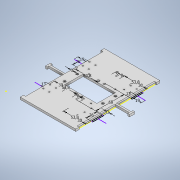
# Autodesk Inventor part: maze_03
Saved by Autodesk Inventor 2020 (Build 240168000, 168)
## iProperties
Created: 2022-07-14
Part Number: maze_03
Material: Типовые
Document SubType Name: Modeling
Designer: akapu
Density: 1 g/cm^3
Appearance: По умолчанию
Author: akapu
Autodesk Inventor part; units mm, degrees
ref_plane "YZ Plane" through (0, 0, 0) normal (1, 0, 0) x (0, 1, 0)
ref_plane "XZ Plane" through (0, 0, 0) normal (0, 1, 0) x (-1, 0, 0)
ref_plane "XY Plane" through (0, 0, 0) normal (0, 0, 1) x (1, 0, 0)
sketch "Эскиз2" plane through (0, 0, 0) normal (0, 1, 0) x (-1, 0, 0)
  line L0 (-166, 0) -> (-166, -200)
  line L1 (-34, 0) -> (-34, -200)
  line L2 (-34, -8) -> (-34, -4)
  line L3 (-9, -53) -> (-196, -53)
  line L4 (-9, -147) -> (-196, -147)
  line L5 (-37, -8) -> (-37, -98)
  line L6 (-37, -98) -> (-29, -98)
  line L7 (-29, -102) -> (-37, -102)
  line L8 (-37, -102) -> (-37, -192)
  line L9 (-166, -192) -> (-163, -192)
  line L10 (-163, -192) -> (-163, -102)
  line L11 (-163, -102) -> (-166, -102)
  line L12 (-166, -102) -> (-166, -192)
  line L13 (-166, -8) -> (-163, -8)
  line L14 (-163, -8) -> (-163, -98)
  line L15 (-163, -98) -> (-166, -98)
  line L16 (-166, -98) -> (-166, -8)
  line L17 (-166, -98) -> (-196, -98)
  line L18 (-196, -98) -> (-196, -102)
  line L19 (-196, -102) -> (-166, -102)
  line L20 (-166, -102) -> (-166, -98)
  line L21 (-29, -98) -> (-4, -98)
  line L22 (-4, -98) -> (-4, -102)
  line L23 (-4, -102) -> (-29, -102)
  line L24 (-29, -102) -> (-29, -98)
  line L25 (-37, -192) -> (-34, -192)
  line L26 (-37, -8) -> (-34, -8)
  line L27 (-4, -102) -> (-4, -106)
  line L28 (-196, -102) -> (-196, -106)
  line L29 (-4, -106) -> (0, -106)
  line L30 (0, -106) -> (0, -94)
  line L31 (0, -94) -> (-4, -94)
  line L32 (-4, -94) -> (-4, -106)
  line L33 (-196, -106) -> (-200, -106)
  line L34 (-200, -106) -> (-200, -94)
  line L35 (-200, -94) -> (-196, -94)
  line L36 (-196, -94) -> (-196, -106)
  line L37 (-34, -200) -> (-166, -200)
  line L38 (-166, 0) -> (-34, 0)
  point P0 (-34, -102)
  point P1 (-34, -98)
  point P2 (-4, -98)
  dimension "d25" = 8
  dimension "d27" = 3
  dimension "d145" = 4
  dimension "d146" = 12
  constraints: 78 end point, 14 parallel, 9 perpendicular, 7 horizontal, 7 point on line, 2 vertical
  measures "d25" distance of L6.end L5.end
  measures "d27" distance of L11.end L10.end
  measures "d145" distance of L22.end L27.end
  measures "d146" distance of L30.end L29.end
extrude "Выдавливание1" add sketch "Эскиз2" along normal blind 5 contours L38 L1 L26 L5 L3 L14 L13 L0 | L15 L14 L3 L5 L6 L1 L7 L8 L4 L10 L11 L0 | L0 L19 L18 L17 | L18 L28 L33 L34 L35 L36 | L6 L24 L7 L1 | L9 L10 L4 L8 L25 L1 L37 L0 | L21 L22 L23 L24 | L32 L31 L30 L29 L27 L22
sketch "Эскиз3" plane through (0, 5, 0) normal (0, 1, 0) x (1, 0, 0)
  line L0 (37, 192) -> (37, 102) projected
  line L1 (37, 147) -> (163, 147)
  line L2 (163, 102) -> (163, 192) projected
  line L3 (37, 98) -> (37, 8) projected
  line L4 (37, 53) -> (163, 53)
  line L5 (163, 147) -> (156, 147)
  line L6 (156, 147) -> (142, 147)
  line L7 (142, 147) -> (142, 155)
  line L8 (142, 155) -> (156, 155)
  line L9 (156, 155) -> (156, 139)
  line L10 (156, 139) -> (142, 139)
  line L11 (142, 139) -> (142, 155)
  line L12 (37, 147) -> (44, 147)
  line L13 (44, 147) -> (58, 147)
  line L14 (58, 147) -> (58, 155)
  line L15 (58, 155) -> (44, 155)
  line L16 (44, 155) -> (44, 139)
  line L17 (44, 139) -> (58, 139)
  line L18 (58, 139) -> (58, 155)
  line L19 (163, 53) -> (156, 53)
  line L20 (156, 53) -> (142, 53)
  line L21 (142, 53) -> (142, 61)
  line L22 (142, 61) -> (58, 61)
  line L23 (58, 61) -> (44, 61)
  line L24 (44, 61) -> (44, 45)
  line L25 (44, 45) -> (58, 45)
  line L26 (58, 45) -> (58, 61)
  line L27 (142, 61) -> (156, 61)
  line L28 (156, 61) -> (156, 45)
  line L29 (156, 45) -> (142, 45)
  line L30 (142, 45) -> (142, 61)
  circle A0 centre (156, 61) radius 1.5
  circle A1 centre (156, 45) radius 1.5
  circle A2 centre (142, 45) radius 1.5
  circle A3 centre (142, 61) radius 1.5
  circle A4 centre (58, 61) radius 1.5
  circle A5 centre (58, 45) radius 1.5
  circle A6 centre (44, 61) radius 1.5
  circle A7 centre (44, 45) radius 1.5
  circle A8 centre (142, 139) radius 1.5
  circle A9 centre (156, 139) radius 1.5
  circle A10 centre (156, 155) radius 1.5
  circle A11 centre (142, 155) radius 1.5
  circle A12 centre (58, 155) radius 1.5
  circle A13 centre (44, 155) radius 1.5
  circle A14 centre (58, 139) radius 1.5
  circle A15 centre (44, 139) radius 1.5
  point P0 (0, 0)
  point P1 (142, 46.5)
  point P2 (143.5, 45)
  dimension "d30" = 7
  dimension "d31" = 14
  dimension "d32" = 8
  dimension "d33" = 16
  dimension "d34" = 7
  dimension "d35" = 14
  dimension "d36" = 8
  dimension "d37" = 16
  dimension "d38" = 7
  dimension "d39" = 14
  dimension "d40" = 8
  dimension "d41" = 16
  dimension "d42" = 16
  dimension "d43" = 3
  dimension "d44" = 3
  dimension "d45" = 3
  dimension "d46" = 3
  dimension "d47" = 3
  dimension "d48" = 3
  dimension "d49" = 3
  dimension "d50" = 3
  dimension "d51" = 3
  dimension "d52" = 3
  dimension "d53" = 3
  dimension "d54" = 3
  dimension "d55" = 3
  dimension "d56" = 3
  dimension "d57" = 3
  dimension "d58" = 3
  constraints: 56 end point, 16 centre point, 16 coincident, 8 parallel, 8 perpendicular, 6 point on line, 5 horizontal, 3 midpoint
  measures "d30" distance of L1.end L5.end
  measures "d31" distance of L5.end L6.end
  measures "d32" distance of L6.end L7.end
  measures "d33" distance of L8.end L9.end
  measures "d34" distance of L1.start L12.end
  measures "d35" distance of L12.end L13.end
  measures "d36" distance of L13.end L14.end
  measures "d37" distance of L16.end L15.end
  measures "d38" distance of L4.end L19.end
  measures "d39" distance of L19.end L20.end
  measures "d40" distance of L20.end L21.end
  measures "d41" distance of L24.end L23.end
  measures "d42" distance of L27.end L28.end
  measures "d43" diameter of A0
  measures "d44" diameter of A1
  measures "d45" diameter of A2
  measures "d46" diameter of A3
  measures "d47" diameter of A4
  measures "d48" diameter of A5
  measures "d49" diameter of A6
  measures "d50" diameter of A7
  measures "d51" diameter of A8
  measures "d52" diameter of A9
  measures "d53" diameter of A10
  measures "d54" diameter of A11
  measures "d55" diameter of A12
  measures "d56" diameter of A13
  measures "d57" diameter of A14
  measures "d58" diameter of A15
extrude "Выдавливание2" cut sketch "Эскиз3" against normal blind 5 contours A13 L15 L16 | L16 L15 A13 | A15 L17 L16 | L16 L17 A15 | A12 L15 L14 | L14 L15 A12 | A14 L17 L18 | L18 L17 A14 | A11 L8 L7 | L7 L8 A11 | A8 L10 L11 | L11 L10 A8 | A10 L8 L9 | L9 L8 A10 | A9 L10 L9 | L9 L10 A9 | A3 L22 L21 | L21 L27 A3 | A2 L29 L30 | L30 L29 A2 | A0 L27 L28 | L28 L27 A0 | A1 L29 L28 | L28 L29 A1 | A5 L25 L26 | L26 L25 A5 | A4 L23 L26 | L26 L22 A4 | L22 A3 L27 | A6 L23 L24 | L24 L23 A6 | A7 L25 L24 | L24 L25 A7 | L23 A4 L22
fillet "Сопряжение1" radius 2 4 edges at (163, 5, -53) (163, 5, -147) (37, 5, -147) (37, 5, -53)
sketch "Эскиз4" plane through (0, 0, 0) normal (0, -1, 0) x (1, 0, 0)
  circle A0 centre (156, -45) radius 1.5 projected
  circle A1 centre (142, -61) radius 1.5 projected
  line L0 (156, -45) -> (142, -45)
  line L1 (142, -45) -> (142, -61)
  line L2 (142, -61) -> (156, -61)
  line L3 (156, -61) -> (156, -45)
  circle A2 centre (156, -139) radius 1.5 projected
  circle A3 centre (142, -155) radius 1.5 projected
  line L4 (156, -139) -> (142, -139)
  line L5 (142, -139) -> (142, -155)
  line L6 (142, -155) -> (156, -155)
  line L7 (156, -155) -> (156, -139)
  circle A4 centre (58, -139) radius 1.5 projected
  circle A5 centre (44, -155) radius 1.5 projected
  line L8 (58, -139) -> (44, -139)
  line L9 (44, -139) -> (44, -155)
  line L10 (44, -155) -> (58, -155)
  line L11 (58, -155) -> (58, -139)
  circle A6 centre (58, -45) radius 1.5 projected
  circle A7 centre (44, -61) radius 1.5 projected
  line L12 (58, -45) -> (44, -45)
  line L13 (44, -45) -> (44, -61)
  line L14 (44, -61) -> (58, -61)
  line L15 (58, -61) -> (58, -45)
  line L16 (37, -98) -> (37, -8) projected
  line L17 (37, -53) -> (37, -66)
  line L18 (163, -8) -> (163, -98) projected
  line L19 (163, -102) -> (163, -192) projected
  line L20 (163, -147) -> (163, -134)
  line L21 (37, -134) -> (37, -160)
  line L22 (37, -192) -> (37, -102) projected
  line L23 (163, -66) -> (163, -40)
  line L24 (37, -40) -> (67, -40)
  line L25 (67, -40) -> (67, -66)
  line L26 (67, -66) -> (37, -66)
  line L27 (37, -66) -> (37, -40)
  line L28 (163, -66) -> (133, -66)
  line L29 (133, -66) -> (133, -40)
  line L30 (133, -40) -> (163, -40)
  line L31 (163, -40) -> (163, -66)
  line L32 (163, -134) -> (133, -134)
  line L33 (133, -134) -> (133, -160)
  line L34 (133, -160) -> (163, -160)
  line L35 (163, -160) -> (163, -134)
  line L36 (37, -134) -> (67, -134)
  line L37 (67, -134) -> (67, -160)
  line L38 (67, -160) -> (37, -160)
  line L39 (37, -160) -> (37, -134)
  line L40 (37, -160) -> (34, -160)
  line L41 (34, -160) -> (34, -134)
  line L42 (34, -134) -> (37, -134)
  line L43 (37, -134) -> (37, -160)
  line L44 (37, -66) -> (34, -66)
  line L45 (34, -66) -> (34, -40)
  line L46 (34, -40) -> (37, -40)
  line L47 (37, -40) -> (37, -66)
  line L48 (163, -40) -> (166, -40)
  line L49 (166, -40) -> (166, -66)
  line L50 (166, -66) -> (163, -66)
  line L51 (163, -66) -> (163, -40)
  line L52 (163, -134) -> (166, -134)
  line L53 (166, -134) -> (166, -160)
  line L54 (166, -160) -> (163, -160)
  line L55 (163, -160) -> (163, -134)
  line L56 (163, -66) -> (109.2, -66)
  line L57 (109.2, -66) -> (109.2, -40)
  line L58 (109.2, -40) -> (163, -40)
  line L59 (163, -40) -> (163, -66)
  line L60 (37, -40) -> (90.8, -40)
  line L61 (90.8, -40) -> (90.8, -66)
  line L62 (90.8, -66) -> (37, -66)
  line L63 (37, -66) -> (37, -40)
  line L64 (163, -134) -> (109.2, -134)
  line L65 (109.2, -134) -> (109.2, -160)
  line L66 (109.2, -160) -> (163, -160)
  line L67 (163, -160) -> (163, -134)
  line L68 (37, -160) -> (90.8, -160)
  line L69 (90.8, -160) -> (90.8, -134)
  line L70 (90.8, -134) -> (37, -134)
  line L71 (37, -134) -> (37, -160)
  line L72 (109.2, -40) -> (101.2, -40)
  line L73 (101.2, -40) -> (101.2, -66)
  line L74 (101.2, -66) -> (109.2, -66)
  line L75 (109.2, -66) -> (109.2, -40)
  line L76 (90.8, -40) -> (98.8, -40)
  line L77 (98.8, -40) -> (98.8, -66)
  line L78 (98.8, -66) -> (90.8, -66)
  line L79 (90.8, -66) -> (90.8, -40)
  line L80 (109.2, -134) -> (101.2, -134)
  line L81 (101.2, -134) -> (101.2, -160)
  line L82 (101.2, -160) -> (109.2, -160)
  line L83 (109.2, -160) -> (109.2, -134)
  line L84 (90.8, -134) -> (98.8, -134)
  line L85 (98.8, -134) -> (98.8, -160)
  line L86 (98.8, -160) -> (90.8, -160)
  line L87 (90.8, -160) -> (90.8, -134)
  line L88 (166, -147) -> (185, -147)
  line L89 (34, -147) -> (15, -147)
  line L90 (34, -53) -> (15, -53)
  line L91 (166, -53) -> (185, -53)
  point P0 (0, 0)
  dimension "d62" = 13
  dimension "d63" = 13
  dimension "d64" = 26
  dimension "d65" = 26
  dimension "d66" = 30
  dimension "d67" = 30
  dimension "d68" = 30
  dimension "d69" = 3
  dimension "d70" = 3
  dimension "d71" = 53.8
  dimension "d72" = 53.8
  dimension "d73" = 53.8
  dimension "d74" = 53.8
  dimension "d75" = 8
  dimension "d76" = 8
  dimension "d77" = 8
  dimension "d78" = 8
  dimension "d93" = 19
  dimension "d94" = 19
  dimension "d95" = 68
  constraints: 176 end point, 40 parallel, 24 horizontal, 20 perpendicular, 16 point on line, 6 midpoint
  measures "d62" distance of L17.start L17.end
  measures "d63" distance of L20.start L20.end
  measures "d64" distance of L21.start L21.end
  measures "d65" distance of L23.start L23.end
  measures "d66" distance of L25.end L26.end
  measures "d67" distance of L29.end L30.end
  measures "d68" distance of L34.end L33.end
  measures "d69" distance of L41.end L42.end
  measures "d70" distance of L49.end L50.end
  measures "d71" distance of L57.end L58.end
  measures "d72" distance of L61.end L62.end
  measures "d73" distance of L66.end L65.end
  measures "d74" distance of L70.end L69.end
  measures "d75" distance of L74.end L73.end
  measures "d76" distance of L77.end L78.end
  measures "d77" distance of L82.end L81.end
  measures "d78" distance of L85.end L86.end
  measures "d93" distance of L88.start L88.end
  measures "d94" distance of L89.start L89.end
  measures "d95" distance of L73.end L80.end
sketch "Эскиз5" plane through (0, 0, 0) normal (0, -1, 0) x (1, 0, 0)
  line L0 (163, -8) -> (163, -98) projected
  line L1 (163, -53) -> (107, -53)
  line L2 (107, -53) -> (107, -147)
  line L3 (107, -147) -> (163, -147)
  line L4 (163, -147) -> (163, -53)
  line L5 (37, -98) -> (37, -8) projected
  line L6 (37, -53) -> (93, -53)
  line L7 (93, -53) -> (93, -147)
  line L8 (93, -147) -> (37, -147)
  line L9 (37, -147) -> (37, -53)
  line L10 (107, -147) -> (93, -147)
  line L11 (93, -147) -> (93, -127)
  line L12 (93, -127) -> (107, -127)
  line L13 (107, -127) -> (107, -147)
  line L14 (107, -53) -> (93, -53)
  line L15 (93, -53) -> (93, -73)
  line L16 (93, -73) -> (107, -73)
  line L17 (107, -73) -> (107, -53)
  circle A0 centre (93, -127) radius 2.5
  circle A1 centre (107, -127) radius 2.5
  circle A2 centre (107, -73) radius 2.5
  circle A3 centre (93, -73) radius 2.5
  point P0 (0, 0)
  dimension "d79" = 56
  dimension "d80" = 56
  dimension "d81" = 20
  dimension "d82" = 20
  dimension "d89" = 5
  dimension "d90" = 5
  dimension "d91" = 5
  dimension "d92" = 5
  constraints: 32 end point, 8 parallel, 4 centre point, 4 coincident, 4 horizontal, 4 perpendicular, 3 point on line, 2 midpoint
  measures "d79" distance of L3.end L2.end
  measures "d80" distance of L7.end L8.end
  measures "d81" distance of L10.end L11.end
  measures "d82" distance of L15.end L14.end
  measures "d89" diameter of A0
  measures "d90" diameter of A1
  measures "d91" diameter of A2
  measures "d92" diameter of A3
extrude "Выдавливание3" cut sketch "Эскиз5" against normal blind 5 contours A2 L2 | L2 L16 A2 | L2 A2 L16 | A3 L16 L7 | L7 A3 | A1 L12 L2 | L2 A1 | A3 L7 L16 | L12 A1 L2 | A0 L7 | L7 L12 A0 | A0 L12 L7
sketch "Эскиз6" plane through (0, 0, 0) normal (0, -1, 0) x (1, 0, 0)
  circle A0 centre (107, -73) radius 2.5 projected
  circle A1 centre (93, -127) radius 2.5 projected
  line L0 (107, -100) -> (93, -100)
  line L1 (100, -100) -> (67.5, -100)
  line L2 (67.5, -100) -> (132.5, -100)
  line L3 (132.5, -100) -> (132.5, -82)
  line L4 (132.5, -82) -> (67.5, -82)
  line L5 (67.5, -82) -> (67.5, -100)
  line L6 (132.5, -100) -> (67.5, -100)
  line L7 (67.5, -100) -> (67.5, -118)
  line L8 (67.5, -118) -> (132.5, -118)
  line L9 (132.5, -118) -> (132.5, -100)
  line L10 (61.5, -82) -> (61.5, -78)
  line L11 (61.5, -78) -> (67.5, -78)
  line L12 (61.5, -78) -> (138.5, -78)
  line L13 (138.5, -78) -> (138.5, -122)
  line L14 (138.5, -122) -> (61.5, -122)
  line L15 (61.5, -122) -> (61.5, -78)
  point P0 (0, 0)
  dimension "d97" = 65
  dimension "d100" = 6
  dimension "d101" = 4
  dimension "d102" = 77
  dimension "d103" = 44
  constraints: 32 end point, 6 parallel, 4 horizontal, 3 perpendicular, 1 midpoint, 1 point on line
  measures "d97" distance of L4.end L3.end
  measures "d100" distance of L10.end L11.end
  measures "d101" distance of L10.start L10.end
  measures "d102" distance of L13.end L14.end
  measures "d103" distance of L12.end L13.end
extrude "Выдавливание5" cut sketch "Эскиз6" against normal blind 5 contours L2 L9 L8 L7 L1 L0 | L0 L1 L5 L4 L3 L2 | L10 L11 L12 L13 L14 L15
sketch "Эскиз7" plane through (0, 5, 0) normal (0, 1, 0) x (1, 0, 0)
  line L0 (138.5, 78) -> (138.5, 122) projected
  line L1 (145.5, 85) -> (54.5, 85)
  line L2 (54.5, 85) -> (54.5, 115)
  line L3 (54.5, 115) -> (145.5, 115)
  line L4 (145.5, 115) -> (145.5, 85)
  line L5 (145.5, 85) -> (142.9, 85)
  line L6 (54.5, 115) -> (57.1, 115)
  line L7 (57.1, 115) -> (142.9, 115)
  line L8 (142.9, 115) -> (142.9, 85)
  line L9 (142.9, 85) -> (57.1, 85)
  line L10 (57.1, 85) -> (57.1, 115)
  line L11 (142.9, 86.5011) -> (145.5, 88.0022)
  line L12 (145.5, 88.0022) -> (148.1, 86.5011)
  line L13 (148.1, 86.5011) -> (148.1, 83.4989)
  line L14 (148.1, 83.4989) -> (145.5, 81.9978)
  line L15 (145.5, 81.9978) -> (142.9, 83.4989)
  line L16 (142.9, 83.4989) -> (142.9, 86.5011)
  line L17 (142.9, 116.5011) -> (145.5, 118.0022)
  line L18 (145.5, 118.0022) -> (148.1, 116.5011)
  line L19 (148.1, 116.5011) -> (148.1, 113.4989)
  line L20 (148.1, 113.4989) -> (145.5, 111.9978)
  line L21 (145.5, 111.9978) -> (142.9, 113.4989)
  line L22 (142.9, 113.4989) -> (142.9, 116.5011)
  line L23 (57.1, 113.4989) -> (54.5, 111.9978)
  line L24 (54.5, 111.9978) -> (51.9, 113.4989)
  line L25 (51.9, 113.4989) -> (51.9, 116.5011)
  line L26 (51.9, 116.5011) -> (54.5, 118.0022)
  line L27 (54.5, 118.0022) -> (57.1, 116.5011)
  line L28 (57.1, 116.5011) -> (57.1, 113.4989)
  line L29 (57.1, 83.4989) -> (54.5, 81.9978)
  line L30 (54.5, 81.9978) -> (51.9, 83.4989)
  line L31 (51.9, 83.4989) -> (51.9, 86.5011)
  line L32 (51.9, 86.5011) -> (54.5, 88.0022)
  line L33 (54.5, 88.0022) -> (57.1, 86.5011)
  line L34 (57.1, 86.5011) -> (57.1, 83.4989)
  circle A0 centre (145.5, 115) radius 1.6
  circle A1 centre (145.5, 85) radius 1.6
  circle A2 centre (54.5, 115) radius 1.6
  circle A3 centre (54.5, 85) radius 1.6
  point P0 (0, 0)
  dimension "d116" = 91
  dimension "d117" = 30
  dimension "d118" = 2.6
  dimension "d119" = 2.6
  dimension "d120" = 3.2
  dimension "d121" = 3.2
  dimension "d122" = 3.2
  dimension "d123" = 3.2
  constraints: 68 end point, 8 coincident, 4 centre point, 4 midpoint, 4 parallel, 2 horizontal, 2 perpendicular, 2 point on line, 52 other
  measures "d116" distance of L2.end L3.end
  measures "d117" distance of L1.end L2.end
  measures "d118" distance of L1.start L5.end
  measures "d119" distance of L2.end L6.end
  measures "d120" diameter of A0
  measures "d121" diameter of A1
  measures "d122" diameter of A2
  measures "d123" diameter of A3
extrude "Выдавливание6" cut sketch "Эскиз7" against normal blind 2 contours L8 L11 L4 A1 L1 | L1 A1 L4 L12 L13 L14 L15 L16 | L34 L29 L30 L31 L32 L2 A3 L1 | L1 A3 L2 L33 L10 | L10 L23 L2 A2 L3 | L3 A2 L2 L24 L25 L26 L27 L28 | L22 L17 L18 L19 L20 L4 A0 L3 | L3 A0 L4 L21 L8
sketch "Эскиз8" plane through (54.5, 5, -115) normal (0, 1, 0) x (1, 0, 0)
  circle A0 centre (91, 0) radius 1.6 projected
  circle A1 centre (91, 0) radius 1.6
  circle A2 centre (91, -30) radius 1.6 projected
  circle A3 centre (91, -30) radius 1.6
  circle A4 centre (0, -30) radius 1.6 projected
  circle A5 centre (0, -30) radius 1.6
  circle A6 centre (0, 0) radius 1.6 projected
  circle A7 centre (0, 0) radius 1.6
  point P0 (-54.5, -115)
  constraints: 4 centre point, 4 coincident
extrude "Выдавливание7" cut sketch "Эскиз8" against normal blind 5
sketch "Эскиз9" plane through (0, 5, 0) normal (0, 1, 0) x (1, 0, 0)
  line L0 (138.5, 122) -> (61.5, 122) projected
  line L1 (61.5, 122) -> (68.5, 122)
  line L2 (61.5, 78) -> (138.5, 78) projected
  line L3 (68.5, 122) -> (68.5, 129)
  line L4 (68.5, 129) -> (131.5, 129)
  line L5 (131.5, 129) -> (131.5, 71)
  line L6 (131.5, 71) -> (68.5, 71)
  line L7 (68.5, 71) -> (68.5, 129)
  circle A0 centre (68.5, 129) radius 1.6
  circle A1 centre (131.5, 129) radius 1.6
  circle A2 centre (131.5, 71) radius 1.6
  circle A3 centre (68.5, 71) radius 1.6
  point P0 (0, 0)
  dimension "d138" = 7
  dimension "d139" = 63
  dimension "d140" = 58
  dimension "d141" = 3.2
  dimension "d142" = 3.2
  dimension "d143" = 3.2
  dimension "d144" = 3.2
  constraints: 12 end point, 4 centre point, 4 coincident, 2 parallel, 1 horizontal, 1 perpendicular, 1 point on line, 1 vertical
  measures "d138" distance of L1.end L3.end
  measures "d139" distance of L5.end L6.end
  measures "d140" distance of L4.end L5.end
  measures "d141" diameter of A0
  measures "d142" diameter of A1
  measures "d143" diameter of A2
  measures "d144" diameter of A3
extrude "Выдавливание8" cut sketch "Эскиз9" against normal blind 10 contours A1 L4 L5 | L5 L4 A1 | A0 L4 L3 | L3 L4 A0 | A2 L6 L5 | L5 L6 A2 | A3 L6 L7 | L7 L6 A3
